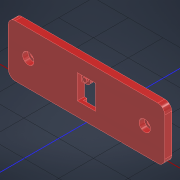
# Autodesk Inventor part: BMP280_Holder
Saved by Autodesk Inventor 2022 (Build 260153000, 153)
## iProperties
Created: 2022-02-02
Part Number: BMP280_Holder
Material: Generisch
Document SubType Name: Modeling
Designer: sleib
Density: 1 g/cm^3
Appearance: Rot
Author: sleib
Autodesk Inventor part; units mm, degrees
ref_plane "YZ Plane" through (0, 0, 0) normal (1, 0, 0) x (0, 1, 0)
ref_plane "XZ Plane" through (0, 0, 0) normal (0, 1, 0) x (-1, 0, 0)
ref_plane "XY Plane" through (0, 0, 0) normal (0, 0, 1) x (1, 0, 0)
sketch "Skizze1" plane through (0, 0, 0) normal (0, 0, 1) x (1, 0, 0)
  line L0 (-45, -15) -> (45, -15)
  line L1 (45, -15) -> (45, 15)
  line L2 (45, 15) -> (-45, 15)
  line L3 (-45, 15) -> (-45, -15)
  line L4 (-45, -15) -> (45, 15) construction
  line L5 (45, -15) -> (-45, 15) construction
  circle A0 centre (-33.4649, 0) radius 1.5
  circle A1 centre (33.4649, 0) radius 1.5
  line L6 (0, -21) -> (0, 21) construction
  line L7 (-63, 0) -> (63, 0) construction
  line L8 (-5.25, 7) -> (5.25, 7)
  line L9 (5.25, 7) -> (5.25, -7)
  line L10 (5.25, -7) -> (-5.25, -7)
  line L11 (-5.25, -7) -> (-5.25, 7)
  circle A2 centre (-2.6, 3.85) radius 1.65 construction
  circle A3 centre (-2.6, 3.85) radius 1.25
  circle A4 centre (-2.6, 3.85) radius 2.5
  line L12 (-5.25, 1.35) -> (-2.6, 1.35)
  line L13 (-0.1, 3.85) -> (-0.1, 7)
  line L14 (-5.25, 1.35) -> (-5.25, 7)
  line L15 (-5.25, 7) -> (-0.1, 7)
  line L16 (-3.75, -15) -> (3.75, -15)
  line L17 (3.75, -15) -> (3.75, -7)
  line L18 (3.75, -7) -> (-3.75, -7)
  line L19 (-3.75, -7) -> (-3.75, -15)
  point P0 (0, 0)
  point P1 (0, -7)
  point P2 (-5.25, -15)
  point P3 (-5.25, -4.15)
  point P4 (5.25, 0)
  point P5 (0, -15)
  dimension "d0" = 66.9299
  dimension "d1" = 30
  dimension "d2" = 90
  dimension "d3" = 3
  dimension "d6" = 14
  dimension "d7" = 10.5
  dimension "d8" = 1
  dimension "d9" = 1.5
  dimension "d10" = 3.3
  dimension "d11" = 2.5
  dimension "d16" = 5
  dimension "d18" = 7.5
  constraints: 36 end point, 8 point on line, 6 parallel, 5 centre point, 5 midpoint, 4 horizontal, 4 perpendicular, 2 coincident, 2 collinear, 2 point on circle, 2 tangent, 1 other
  measures "d0" distance of A1.centre A0.centre
  measures "d1" distance of L2.end L0.start
  measures "d2" distance of L1.end L2.end
  measures "d3" diameter of A0
  measures "d6" distance of L10.end L8.start
  measures "d7" distance between parallel lines of L9 L11
  measures "d8" distance edge to line of A2 L11
  measures "d9" distance edge to line of A2 L8
  measures "d10" diameter of A2
  measures "d11" diameter of A3
  measures "d16" diameter of A4
  measures "d18" distance between parallel lines of L17 L19
extrude "Extrusion2" add sketch "Skizze1" along normal blind 4 contours L3 L2 L1 L0 L17 L10 L9 L8 L11 L19 | L19 L10 L17 L0
extrude "Extrusion3" add sketch "Skizze1" along normal blind 1.5 contours L11 L8 L13 A4 L12 | A4
extrude "Extrusion6" cut sketch "Skizze1" along normal blind 2 contours L19 L10 L17 L0
fillet "Rundung1" radius 4 4 edges at (-45, -15, 2) (-45, 15, 2) (45, 15, 2) (45, -15, 2)
sketch "Skizze2" plane through (0, 0, 4) normal (0, 0, 1) x (1, 0, 0)
  circle A0 centre (-33.4649, 0) radius 1.5 projected
  circle A1 centre (33.4649, 0) radius 1.5 projected
  point P0 (0, 0)
  point P1 (32.8585, 1.3744)
  constraints: 2 coincident
hole "Bohrung1" at (-33.4649, 0, 4) at (33.4649, 0, 4) direction (0, 0, -1) diameter 3.4 end through all counterbore diameter 6.5 counterbore depth 3 clearance for "Inbusschraube DIN EN ISO 4762" size "M3" standard "DIN"
extrude "Extrusion7" add sketch "Skizze1" along normal blind 2.5 contours A3
